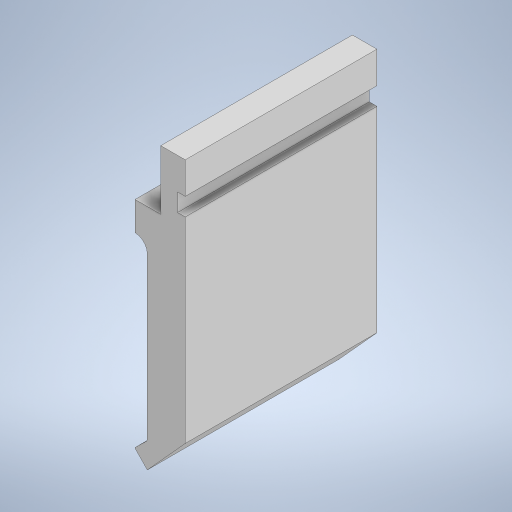
# Autodesk Inventor part: Knife
Saved by Autodesk Inventor 2023.1 (Build 271208000, 208)
## iProperties
Created: 2023-11-13
Part Number: Knife
Material: Generic
Document SubType Name: Modeling
Designer: admin
Density: 1 g/cm^3
Appearance: Default
Author: admin
Autodesk Inventor part; units mm, degrees
ref_plane "YZ Plane" through (0, 0, 0) normal (1, 0, 0) x (0, 1, 0)
ref_plane "XZ Plane" through (0, 0, 0) normal (0, 1, 0) x (-1, 0, 0)
ref_plane "XY Plane" through (0, 0, 0) normal (0, 0, 1) x (1, 0, 0)
sketch "Sketch1" plane through (0, 0, 0) normal (0, 0, 1) x (1, 0, 0)
  line L0 (0, 0) -> (19.8, 21.868)
  line L1 (0, 0) -> (-6.2796, 6.4472)
  arc A0 (-6.2717, 7.0475) -> (-6.2796, 6.4472) centre (-5.9755, 6.7434) ccw
  line L2 (-6.2717, 7.0475) -> (-0.6045, 12.5673)
  line L3 (19.8, 21.868) -> (19.8, 124.2)
  line L4 (19.8, 124.2) -> (15.8, 124.2)
  line L5 (15.8, 124.2) -> (15.8, 133.5)
  line L6 (15.8, 133.5) -> (19.8, 133.5)
  line L7 (19.8, 133.5) -> (19.8, 150)
  line L8 (19.8, 150) -> (7, 150)
  line L9 (7, 150) -> (7, 119)
  line L10 (7, 119) -> (-6.4, 119)
  line L11 (-6.4, 119) -> (-6.4, 104)
  arc A1 (0, 97.6) -> (-6.4, 104) centre (-6.4, 97.6) ccw
  line L12 (0, 97.6) -> (0, 14)
  arc A2 (-0.6045, 12.5673) -> (0, 14) centre (-2, 14) ccw
  line L13 (0, 0) -> (-13.9547, 14.3271) construction
  line L14 (-13.9547, 14.3271) -> (-3.2093, 24.7932) construction
  line L15 (69.4917, 19.7836) -> (93.1308, 37.4314)
  line L16 (93.1308, 37.4314) -> (112.8263, 137.8506)
  line L17 (112.8263, 137.8506) -> (108.9011, 138.6205)
  line L18 (108.9011, 138.6205) -> (110.691, 147.7466)
  line L19 (110.691, 147.7466) -> (114.6162, 146.9767)
  line L20 (114.6162, 146.9767) -> (117.7919, 163.1682)
  line L21 (117.7919, 163.1682) -> (105.2312, 165.6318)
  line L22 (105.2312, 165.6318) -> (99.2648, 135.2114)
  line L23 (99.2648, 135.2114) -> (86.1153, 137.7904)
  line L24 (86.1153, 137.7904) -> (83.2283, 123.0709)
  line L25 (83.2283, 123.0709) -> (88.2769, 115.5587)
  line L26 (88.2769, 115.5587) -> (71.9639, 32.3855)
  line L27 (71.9639, 32.3855) -> (64.4618, 27.4868)
  line L28 (64.4618, 27.4868) -> (69.4917, 19.7836)
  line L29 (71.9639, 32.3855) -> (69.4917, 19.7836) construction
  dimension "d1" = 150
  dimension "d2" = 2
  dimension "d4" = 19.8
  dimension "d5" = 29.5
  dimension "d6" = 26.2
  dimension "d7" = 9
  dimension "d8" = 16.5
  dimension "d9" = 9.3
  dimension "d10" = 12.8
  dimension "d11" = 31
  dimension "d12" = 4
  dimension "d13" = 15
  dimension "d14" = 14
  dimension "d15" = 20
  dimension "d16" = 15
  dimension "d19" = 19.8
  dimension "d20" = 9.2
  dimension "d21" = 150
  dimension "d22" = 16.5
  dimension "d23" = 12.8
  dimension "d24" = 31
  dimension "d25" = 26.2
  dimension "d26" = 135
  dimension "d27" = 15
  dimension "d28" = 4
  dimension "d29" = 29.5
  dimension "d30" = 9.3
  dimension "d31" = 86.4
  dimension "d32" = 42.16
  constraints: 60 end point, 17 perpendicular, 6 point on circle, 6 point on line, 6 tangent, 3 centre point, 2 parallel, 1 vertical, 1 vertical alignment
  measures "d1" distance from line of L0.start L8
  measures "d2" radius of A2
  measures "d4" distance between parallel lines of L3 L12
  measures "d5" distance of L0.start L0.end
  measures "d6" distance between parallel lines of L11 L3
  measures "d7" distance of L0.start L1.end
  measures "d8" distance of L6.end L7.end
  measures "d9" distance of L4.end L5.end
  measures "d10" distance of L7.end L8.end
  measures "d11" distance of L8.end L9.end
  measures "d12" distance of L5.end L6.end
  measures "d13" distance of L10.end L11.end
  measures "d14" distance of L12.end L0.start
  measures "d15" distance of L0.start L13.end
  measures "d16" distance of L13.end L14.end
  measures "d19" distance between parallel lines of L16 L26
  measures "d20" distance of L27.end L15.start
  measures "d21" distance from line of L21 L15.start
  measures "d22" distance of L19.end L20.end
  measures "d23" distance of L20.end L22.start
  measures "d24" distance of L22.start L23.start
  measures "d25" distance between parallel lines of L16 L24
  measures "d26" angle of L24 L25
  measures "d27" distance of L24.start L24.end
  measures "d28" distance of L18.end L19.end
  measures "d29" distance of L15.start L16.start
  measures "d30" distance of L17.end L18.end
  measures "d31" angle of L28 L15
  measures "d32" angle of L15 L26
extrude "Extrusion1" add sketch "Sketch1" along normal blind 100 contours L1 A0 L2 A2 L12 A1 L11 L10 L9 L8 L7 L6 L5 L4 L3 L0
body "Solid1"
